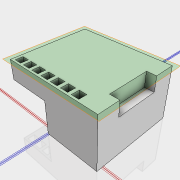
# Autodesk Inventor part: ЛЦМК0000002.00.00.00.00.04
Saved by Autodesk Inventor 2021.2 (Build 252289000, 289)
## iProperties
Created: 2025-10-23
Part Number: ЛЦМК0000002.00.00.00.00.04
Material: Типовые
Document SubType Name: Modeling
Designer: Захаров
Density: 1 g/cm^3
Appearance: По умолчанию
Author: Захаров
Autodesk Inventor part; units mm, degrees
ref_plane "YZ Plane" through (0, 0, 0) normal (1, 0, 0) x (0, 1, 0)
ref_plane "XZ Plane" through (0, 0, 0) normal (0, 1, 0) x (-1, 0, 0)
ref_plane "XY Plane" through (0, 0, 0) normal (0, 0, 1) x (1, 0, 0)
ref_plane "РабПлоскость1" through (1.75, -2.8, -7.7) normal (0, -1, 0) x (1, 0, 0)
sketch "Эскиз1" plane through (1.75, -2.8, -7.7) normal (0, -1, 0) x (1, 0, 0)
  line L0 (-3.35, 6.9) -> (-4.95, 6.9) projected
  line L1 (-4.95, 6.9) -> (-4.95, 8.5) projected
  line L2 (-4.95, 8.5) -> (-3.35, 8.5) projected
  line L3 (-3.35, 8.5) -> (-3.35, 6.9) projected
  line L4 (-8.15, 6.9) -> (-9.75, 6.9) projected
  line L5 (-9.75, 6.9) -> (-9.75, 8.5) projected
  line L6 (-9.75, 8.5) -> (-8.15, 8.5) projected
  line L7 (-8.15, 8.5) -> (-8.15, 6.9) projected
  line L8 (1.45, 6.9) -> (-0.15, 6.9) projected
  line L9 (-0.15, 6.9) -> (-0.15, 8.5) projected
  line L10 (-0.15, 8.5) -> (1.45, 8.5) projected
  line L11 (1.45, 8.5) -> (1.45, 6.9) projected
  line L12 (-0.95, 6.9) -> (-2.55, 6.9) projected
  line L13 (-2.55, 6.9) -> (-2.55, 8.5) projected
  line L14 (-2.55, 8.5) -> (-0.95, 8.5) projected
  line L15 (-0.95, 8.5) -> (-0.95, 6.9) projected
  line L16 (3.85, 6.9) -> (2.25, 6.9) projected
  line L17 (2.25, 6.9) -> (2.25, 8.5) projected
  line L18 (2.25, 8.5) -> (3.85, 8.5) projected
  line L19 (3.85, 8.5) -> (3.85, 6.9) projected
  line L20 (-5.75, 6.9) -> (-7.35, 6.9) projected
  line L21 (-7.35, 6.9) -> (-7.35, 8.5) projected
  line L22 (-7.35, 8.5) -> (-5.75, 8.5) projected
  line L23 (-5.75, 8.5) -> (-5.75, 6.9) projected
  line L24 (6.25, 6.9) -> (4.65, 6.9) projected
  line L25 (4.65, 6.9) -> (4.65, 8.5) projected
  line L26 (4.65, 8.5) -> (6.25, 8.5) projected
  line L27 (6.25, 8.5) -> (6.25, 6.9) projected
  line L28 (8.5, 4.5) -> (10.5, 4.5) projected
  line L29 (10.5, 4.5) -> (10.5, 9) projected
  line L30 (10.5, 9) -> (-10.5, 9) projected
  line L31 (-10.5, 9) -> (-10.5, -9) projected
  line L32 (-10.5, -9) -> (10.5, -9) projected
  line L33 (10.5, -9) -> (10.5, -4.5) projected
  line L34 (10.5, -4.5) -> (8.5, -4.5) projected
  line L35 (8.5, -4.5) -> (8.5, 4.5) projected
  point P0 (-1.75, 7.7)
extrude "Выдавливание1" add sketch "Эскиз1" along normal blind 4.2
sketch "Эскиз2" plane through (1.75, -7, -7.7) normal (0, -1, 0) x (1, 0, 0)
  line L0 (10.5, -9) -> (10.5, -4.5) projected
  line L1 (10.5, 9) -> (-10.5, 9) projected
  line L2 (10.5, -9) -> (-1.5, -9)
  line L3 (-1.5, -9) -> (-1.5, 9)
  line L4 (-1.5, 9) -> (10.5, 9)
  line L5 (10.5, 9) -> (10.5, -9)
  point P0 (-1.75, 7.7)
  dimension "d2" = 12
  constraints: 8 end point, 2 parallel, 1 horizontal, 1 perpendicular, 1 point on line
  measures "d2" distance of L3.end L4.end
extrude "Выдавливание2" add sketch "Эскиз2" along normal blind 7.3
sketch "Эскиз3" plane through (1.75, -14.3, -7.7) normal (0, -1, 0) x (1, 0, 0)
  line L0 (-4.95, 6.9) -> (-3.35, 6.9) projected
  line L1 (-3.35, 6.9) -> (-3.35, 8.5) projected
  line L2 (-3.35, 8.5) -> (-4.95, 8.5) projected
  line L3 (-4.95, 8.5) -> (-4.95, 6.9) projected
  line L4 (-9.75, 6.9) -> (-8.15, 6.9) projected
  line L5 (-8.15, 6.9) -> (-8.15, 8.5) projected
  line L6 (-8.15, 8.5) -> (-9.75, 8.5) projected
  line L7 (-9.75, 8.5) -> (-9.75, 6.9) projected
  line L8 (-0.15, 6.9) -> (1.45, 6.9) projected
  line L9 (1.45, 6.9) -> (1.45, 8.5) projected
  line L10 (1.45, 8.5) -> (-0.15, 8.5) projected
  line L11 (-0.15, 8.5) -> (-0.15, 6.9) projected
  line L12 (-2.55, 6.9) -> (-0.95, 6.9) projected
  line L13 (-0.95, 6.9) -> (-0.95, 8.5) projected
  line L14 (-0.95, 8.5) -> (-2.55, 8.5) projected
  line L15 (-2.55, 8.5) -> (-2.55, 6.9) projected
  line L16 (2.25, 6.9) -> (3.85, 6.9) projected
  line L17 (3.85, 6.9) -> (3.85, 8.5) projected
  line L18 (3.85, 8.5) -> (2.25, 8.5) projected
  line L19 (2.25, 8.5) -> (2.25, 6.9) projected
  line L20 (-7.35, 6.9) -> (-5.75, 6.9) projected
  line L21 (-5.75, 6.9) -> (-5.75, 8.5) projected
  line L22 (-5.75, 8.5) -> (-7.35, 8.5) projected
  line L23 (-7.35, 8.5) -> (-7.35, 6.9) projected
  line L24 (4.65, 6.9) -> (6.25, 6.9) projected
  line L25 (6.25, 6.9) -> (6.25, 8.5) projected
  line L26 (6.25, 8.5) -> (4.65, 8.5) projected
  line L27 (4.65, 8.5) -> (4.65, 6.9) projected
  line L28 (10.5, 9) -> (-10.5, 9) projected
  line L29 (10.5, -9) -> (10.5, 9) projected
  line L30 (-10.5, -9) -> (10.5, -9) projected
  line L31 (-10.5, 9) -> (-10.5, -9) projected
  point P0 (-1.75, 7.7)
extrude "Выдавливание3" cut sketch "Эскиз3" against normal blind 7.3 contours L11 L10 L9 L8 | L15 L14 L13 L12 | L19 L18 L17 L16 | L27 L26 L25 L24
sketch "Эскиз4" plane through (1.75, -7, -7.7) normal (0, 1, 0) x (1, 0, 0)
  line L0 (8.5, -4.5) -> (10.5, -4.5) projected
  line L1 (10.5, 4.5) -> (10.5, -4.5) projected
  line L2 (10.5, 4.5) -> (8.5, 4.5) projected
  line L3 (8.5, 4.5) -> (8.5, -4.5) projected
  point P0 (-1.75, -7.7)
ref_plane "РабПлоскость2" through (10.25, -6, -12.2) normal (0, -1, 0) x (1, 0, 0)
extrude "Выдавливание4" add sketch "Эскиз4" along normal up to surface (1 mm away)
